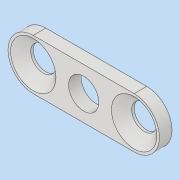
# Autodesk Inventor part: pushSwitchBushingHolderRear
Saved by Autodesk Inventor 2017 (Build 210142000, 142)
## iProperties
Created: 2016-12-03
Part Number: pushSwitchBushingHolderRear
Material: ABS Plastic
Document SubType Name: Modeling
Designer: techn
Density: 1.06 g/cm^3
Appearance: Smooth - White
Author: techn
Autodesk Inventor part; units mm, degrees
ref_plane "YZ Plane" through (0, 0, 0) normal (1, 0, 0) x (0, 1, 0)
ref_plane "XZ Plane" through (0, 0, 0) normal (0, 1, 0) x (-1, 0, 0)
ref_plane "XY Plane" through (0, 0, 0) normal (0, 0, 1) x (1, 0, 0)
sketch "Sketch1" plane through (0, 0, 0) normal (0, 0, 1) x (1, 0, 0)
  circle A0 centre (0, 0) radius 1.905
  line L0 (0, 0) -> (6.35, 0)
  line L1 (6.35, 0) -> (-6.35, 0)
  circle A1 centre (-6.35, 0) radius 1.5875
  circle A2 centre (6.35, 0) radius 1.5875
  line L2 (-9.525, 3.175) -> (9.525, 3.175)
  line L3 (9.525, 3.175) -> (9.525, -3.175)
  line L4 (9.525, -3.175) -> (-9.525, -3.175)
  line L5 (-9.525, -3.175) -> (-9.525, 3.175)
  dimension "d0" = 3.81
  dimension "d1" = 6.35
  dimension "d2" = 12.7
  dimension "d3" = 3.175
  dimension "d4" = 3.175
  dimension "d5" = 19.05
  dimension "d6" = 9.525
  dimension "d7" = 6.35
  dimension "d8" = 3.175
  constraints: 12 end point, 3 centre point, 3 coincident, 2 horizontal, 2 parallel, 1 perpendicular, 1 point on line
  measures "d0" diameter of A0
  measures "d1" distance of L0.start L0.end
  measures "d2" distance of L0.end L1.end
  measures "d3" diameter of A1
  measures "d4" diameter of A2
  measures "d5" distance between parallel lines of L3 L5
  measures "d6" distance from line of L3 point (0, 0)
  measures "d7" distance of L2.end L3.end
  measures "d8" distance from line of L2 point (0, 0)
sketch "Sketch1 outline for Extrusion1" plane through (0, 0, 0) normal (0, 0, 1) x (1, 0, 0)
  line L0 (-9.525, 3.175) -> (9.525, 3.175)
  line L1 (-9.525, -3.175) -> (-9.525, 3.175)
  line L2 (9.525, 3.175) -> (9.525, -3.175)
  line L3 (9.525, -3.175) -> (-9.525, -3.175)
  circle A0 centre (-6.35, 0) radius 1.5875
  circle A1 centre (0, 0) radius 1.905
  circle A2 centre (6.35, 0) radius 1.5875
extrude "Extrusion1" add sketch "Sketch1 outline for Extrusion1" along normal blind 1.5875
chamfer "Chamfer1" distance 1.27 angle 45 2 edges at (-7.9375, 0, 1.5875) (4.7625, 0, 1.5875)
fillet "Fillet1" radius 3.175 4 edges at (-9.525, 3.175, 0.7937) (-9.525, -3.175, 0.7937) (9.525, -3.175, 0.7937) (9.525, 3.175, 0.7937)
body "Solid1"
